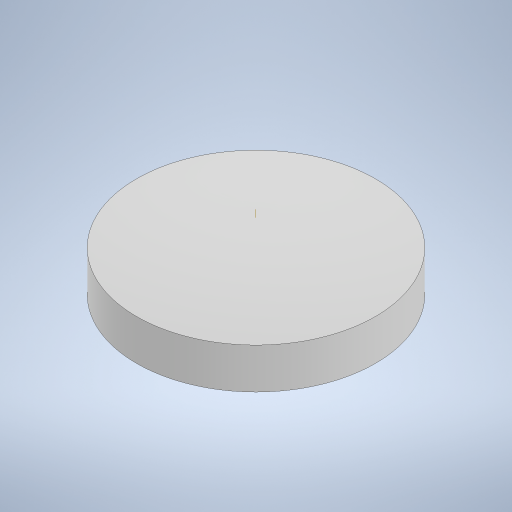
# Autodesk Inventor part: Enemy_turret_collision
Saved by Autodesk Inventor 2024 (Build 280153000, 153)
## iProperties
Created: 2026-05-20
Part Number: Enemy_turret_collision
Material: Generic
Document SubType Name: Modeling
Designer: warny
Density: 1 g/cm^3
Appearance: Default
Author: warny
Autodesk Inventor part; units mm, degrees
ref_plane "YZ Plane" through (0, 0, 0) normal (1, 0, 0) x (0, 1, 0)
ref_plane "XZ Plane" through (0, 0, 0) normal (0, 1, 0) x (-1, 0, 0)
ref_plane "XY Plane" through (0, 0, 0) normal (0, 0, 1) x (1, 0, 0)
sketch "Sketch2" plane through (0, 0, 0) normal (0, 1, 0) x (-1, 0, 0)
  circle A0 centre (0, 0) radius 179.6
  dimension "d0" = 359.2
  constraints: 1 centre point, 1 coincident
  measures "d0" diameter of A0
extrude "Extrusion1" add sketch "Sketch2" along normal blind 61.2
sketch "Sketch3" plane through (0, 0, 0) normal (0, 0, 1) x (1, 0, 0)
  line L0 (179.6, 61.2) -> (-179.6, 61.2) projected
  line L1 (179.6, 61.2) -> (-179.6, 61.2) projected
  line L2 (179.6, 0) -> (-179.6, 0) projected
  line L3 (0, -12.24) -> (0, 73.44) projected
  line L4 (0, 61.2) -> (179.6, 61.2)
  line L5 (0, 61.2) -> (0, 100.6)
  arc A0 (179.6, 61.2) -> (0, 100.6) centre (0, -328.4421) ccw
  point P0 (0, 0)
  point P1 (0, 61.2)
  dimension "d3" = 39.4
  dimension "d4" = 0
  constraints: 4 end point, 2 midpoint, 2 point on circle, 2 point on line, 1 centre point, 1 coincident, 1 collinear, 1 perpendicular
  measures "d3" distance of L5.end L4.start
  measures "d4" distance from line of A0.centre L3
revolve "Revolution1" add sketch "Sketch3" angle 360 about axis through (0, -10, 0) along (0, 1, 0)
body "Solid1"
